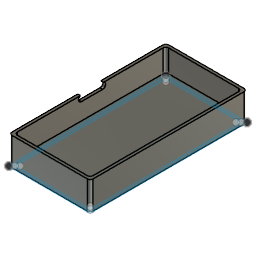
waterbox (Autodesk Fusion 360 design; units mm, degrees)
part number: 2026-07-11-15-02-25-101
Autodesk Fusion 360 part; units mm, degrees
sketch "Sketch1" plane through (0, 0, 0) normal (0, 0, 1) x (1, 0, 0)
  line L0 (-90, 75) -> (180, 75)
  line L1 (190, 65) -> (190, -475)
  line L2 (180, -485) -> (-90, -485)
  line L3 (-100, -475) -> (-100, 65)
  line L4 (170, -475) -> (-80, -475)
  line L5 (-90, -465) -> (-90, 55)
  line L6 (-80, 65) -> (170, 65)
  line L7 (180, 55) -> (180, -465)
  arc A0 (190, 65) -> (180, 75) centre (180, 65) ccw
  arc A1 (180, 55) -> (170, 65) centre (170, 55) ccw
  arc A2 (-80, 65) -> (-90, 55) centre (-80, 55) ccw
  arc A3 (180, -485) -> (190, -475) centre (180, -475) ccw
  arc A4 (-90, 75) -> (-100, 65) centre (-90, 65) ccw
  arc A5 (170, -475) -> (180, -465) centre (170, -465) ccw
  arc A6 (-90, -465) -> (-80, -475) centre (-80, -465) ccw
  arc A7 (-100, -475) -> (-90, -485) centre (-90, -475) ccw
  point P0 (-100, 75)
  point P1 (190, 75)
  point P2 (-100, -485)
  dimension "d1" = 290
  dimension "d2" = 560
  dimension "d4" = 10
  dimension "d5" = 10
  constraint perpendicular L0 L1
  constraint parallel L0 L2
  constraint parallel L1 L3
  constraint horizontal L0
  constraint coincident P1 L0
  constraint coincident P1 L1
  constraint tangent L0 A0
  constraint tangent L1 A0
  constraint tangent L6 A1
  constraint tangent L7 A1
  constraint equal A0 A1
  constraint tangent L5 A2
  constraint tangent L6 A2
  constraint equal A0 A2
  constraint tangent L1 A3
  constraint tangent L2 A3
  constraint equal A0 A3
  constraint coincident P0 L0
  constraint coincident P0 L3
  constraint tangent L0 A4
  constraint tangent L3 A4
  constraint equal A0 A4
  constraint tangent L4 A5
  constraint tangent L7 A5
  constraint equal A0 A5
  constraint tangent L4 A6
  constraint tangent L5 A6
  constraint equal A0 A6
  constraint coincident P2 L2
  constraint coincident P2 L3
  constraint tangent L2 A7
  constraint tangent L3 A7
  measures "d1" distance of P0 P1
  measures "d2" distance of P0 P2
  measures "d4" radius of A0
  measures "d5" radius of A7
extrude "Extrude1" add sketch "Sketch1" along normal blind 100
extrude "Extrude2" add sketch "Sketch1" along normal blind 20 contours L4 L5 L6 L7 A1 A2 A5 A6
sketch "Sketch2" plane through (-100, 0, 0) normal (-1, 0, 0) x (0, -1, 0)
  line L0 (-65, 0) -> (475, 0)
  line L1 (475, 0) -> (475, 100)
  line L2 (475, 100) -> (-65, 100)
  line L3 (-65, 100) -> (-65, 0)
  line L4 (160, 79.717) -> (236.5175, 79.717)
  arc A0 (236.5175, 79.717) -> (236.5175, 100.283) centre (236.5175, 90) ccw
  line L5 (236.5175, 100.283) -> (160, 100.283)
  arc A1 (160, 100.283) -> (160, 79.717) centre (160, 90) ccw
  line L6 (160, 90) -> (236.5175, 90) construction
  constraint tangent L4 A0
  constraint tangent A0 L5
  constraint parallel L4 L5
  constraint tangent L5 A1
  constraint tangent L4 A1
  constraint parallel L2 L6
extrude "Extrude3" cut sketch "Sketch2" against normal blind 40 contours L2 L4 A0 A1
